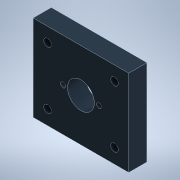
# Autodesk Inventor part: Placa cilindro hidraulico
Saved by Autodesk Inventor 2021 (Build 250183000, 183)
## iProperties
Created: 2021-07-12
Part Number: Placa cilindro hidraulico
Material: Generic
Document SubType Name: Modeling
Designer: Nelson
Density: 1 g/cm^3
Appearance: Default(1)
Author: Nelson
Autodesk Inventor part; units mm, degrees
ref_plane "YZ Plane" through (0, 0, 0) normal (1, 0, 0) x (0, 1, 0)
ref_plane "XZ Plane" through (0, 0, 0) normal (0, 1, 0) x (-1, 0, 0)
ref_plane "XY Plane" through (0, 0, 0) normal (0, 0, 1) x (1, 0, 0)
sketch "Sketch1" plane through (0, 0, 0) normal (0, 0, 1) x (1, 0, 0)
  line L0 (0, 0) -> (200, 0)
  line L1 (0, 180) -> (0, 0)
  line L2 (200, 180) -> (0, 180)
  circle A0 centre (100, 90) radius 28
  circle A1 centre (30, 150) radius 8
  circle A2 centre (170, 150) radius 8
  circle A3 centre (170, 30) radius 8
  circle A4 centre (30, 30) radius 8
  line L3 (200, 0) -> (200, 180)
  dimension "d1" = 56
  dimension "d2" = 70
  dimension "d5" = 60
  dimension "d6" = 70
  dimension "d7" = 60
  dimension "d8" = 70
  dimension "d9" = 70
  dimension "d10" = 60
  dimension "d11" = 60
  dimension "d35" = 180
  dimension "d37" = 200
  dimension "d39" = 16
  dimension "d41" = 30
  dimension "d42" = 30
  constraints: 8 end point, 5 centre point, 3 equal radius, 2 parallel, 1 coincident
  measures "d1" diameter of A0
  measures "d2" horizontal distance of A1.centre A0.centre
  measures "d5" vertical distance of A0.centre A1.centre
  measures "d6" horizontal distance of A0.centre A2.centre
  measures "d7" vertical distance of A0.centre A2.centre
  measures "d8" horizontal distance of A4.centre A0.centre
  measures "d9" horizontal distance of A3.centre A0.centre
  measures "d10" vertical distance of A0.centre A4.centre
  measures "d11" vertical distance of A3.centre A0.centre
  measures "d35" distance of L0.end L2.start
  measures "d37" distance of L2.start L1.start
  measures "d39" diameter of A4
  measures "d41" distance from line of L1 A1.centre
  measures "d42" distance from line of L2 A1.centre
extrude "Extrusion1" add sketch "Sketch1" against normal blind 38
sketch "Sketch2" plane through (0, 0, 0) normal (0, 0, 1) x (1, 0, 0)
  circle A0 centre (100, 90) radius 28 projected
  line L0 (200, 180) -> (0, 180) projected
  line L1 (0, 180) -> (0, 0) projected
  circle A1 centre (30, 30) radius 8 projected
  circle A2 centre (30, 150) radius 8 projected
  circle A3 centre (170, 30) radius 8 projected
  point P0 (137.5, 90)
  point P1 (62.5, 90)
  dimension "d45" = 37.5
  dimension "d46" = 37.5
  dimension "d47" = 60
  dimension "d48" = 60
  measures "d45" distance of point (62.5, 90) A0.centre
  measures "d46" distance of A0.centre point (137.5, 90)
  measures "d47" vertical distance of A3.centre point (137.5, 90)
  measures "d48" vertical distance of A1.centre point (62.5, 90)
hole "Hole1" at (62.5, 90, 0) at (137.5, 90, 0) direction (0, 0, -1) diameter 10.5918 depth 38 thread size "1/2-13 UNC" class "2B" standard "ANSI Unified Screw Threads"
equation "\"d6\" = d2"
equation "\"d7\" = d5"
equation "\"d8\" = d2"
equation "\"d9\" = d2"
equation "\"d10\" = d5"
equation "\"d11\" = d5"
equation "\"d46\" = d45"
equation "\"d48\" = d47"
body "Solid1"
